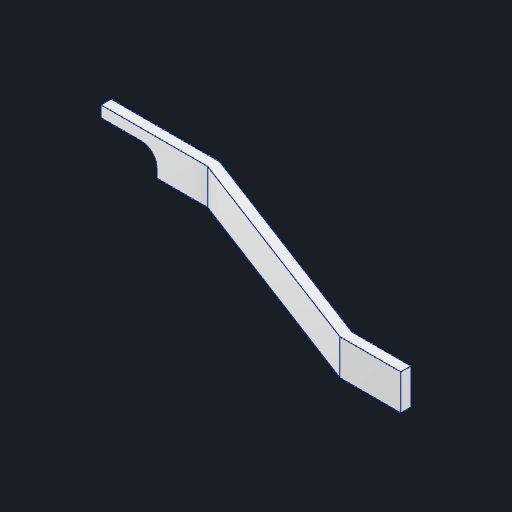
# Autodesk Inventor part: Y_zigZag
Saved by Autodesk Inventor 2024 (Build 280153000, 153)
## iProperties
Created: 2023-06-20
Part Number: Y_zigZag
Material: Aluminum 6061
Document SubType Name: Modeling
Designer: KirikDK
Density: 2.7 g/cm^3
Appearance: Aluminum - Flat
Mass: 2671.61 g
Surface Area: 1326.69 cm^2
Volume: 989.485 cm^3
Author: KirikDK
Autodesk Inventor part; units mm, degrees
ref_plane "YZ Plane" through (0, 0, 0) normal (1, 0, 0) x (0, 1, 0)
ref_plane "XZ Plane" through (0, 0, 0) normal (0, 1, 0) x (-1, 0, 0)
ref_plane "XY Plane" through (0, 0, 0) normal (0, 0, 1) x (1, 0, 0)
sketch "Sketch1" plane through (0, 0, 0) normal (0, 1, 0) x (-1, 0, 0)
  line L0 (-315.9154, 73.2239) -> (-195.9154, 73.2239)
  line L1 (-195.9154, 73.2239) -> (224.0846, -86.7761)
  line L2 (324.0846, -86.7761) -> (224.0846, -86.7761)
  line L3 (324.0846, -106.7761) -> (220.4041, -106.7761)
  line L4 (220.4041, -106.7761) -> (-199.5959, 53.2239)
  line L5 (-199.5959, 53.2239) -> (-315.9154, 53.2239)
  line L6 (324.0846, -106.7761) -> (324.0846, -86.7761)
  line L7 (-315.9154, 53.2239) -> (-315.9154, 73.2239)
  point P0 (0, 0)
  dimension "d2" = 100
  dimension "d3" = 449.4441
  dimension "d4" = 120
  dimension "d5" = 159.146
  dimension "d6" = 159.146
  dimension "d7" = 20
  constraints: 16 end point, 1 horizontal, 1 parallel, 1 vertical, 2 other
  measures "d2" distance of L2.start L1.end
  measures "d3" distance of L0.end L1.end
  measures "d4" distance of L0.start L0.end
  measures "d5" angle of L1 L0
  measures "d6" angle of L2 L1
  measures "d7" distance between parallel lines of L2 L3
extrude "Extrusion1" add sketch "Sketch1" along normal blind 70
sketch "Sketch2" plane through (-324.0846, 0, -106.7761) normal (-1, 0, 0) x (0, 0, 1)
  line L0 (0, 48) -> (20, 48)
  line L1 (20, 48) -> (20, 70)
  line L2 (20, 70) -> (0, 70)
  line L3 (0, 70) -> (0, 48)
  point P0 (106.7761, 0)
  constraints: 8 end point, 2 parallel, 1 horizontal, 1 perpendicular
extrude "Extrusion2" add sketch "Sketch2" along normal blind 110
fillet "Fillet1" radius 30 1 edges at (-324.0846, 48, -96.7761)
body "Solid1"
